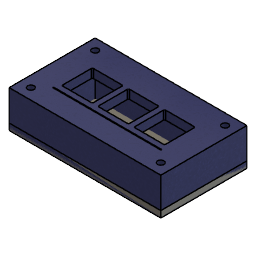
My case (Autodesk Fusion 360 design; units mm, degrees)
part number: 2026-08-28-17-32-42-272
Autodesk Fusion 360 part; units mm, degrees
sketch "Sketch1" plane through (0, 0, 0) normal (0, 1, 0) x (1, 0, 0)
  line L0 (0, 0) -> (49.4, 0)
  line L1 (49.4, 0) -> (49.4, -19.4)
  line L2 (49.4, -19.4) -> (0, -19.4)
  line L3 (0, -19.4) -> (0, 0)
  line L4 (-10, 10) -> (59.4, 10)
  line L5 (59.4, 10) -> (59.4, -29.4)
  line L6 (59.4, -29.4) -> (-10, -29.4)
  line L7 (-10, -29.4) -> (-10, 10)
  circle A0 centre (-5, 5) radius 1.45
  circle A1 centre (54.4, 5) radius 1.45
  circle A2 centre (54.4, -24.4) radius 1.45
  circle A3 centre (-5, -24.4) radius 1.45
  point P0 (-5, 5)
  point P1 (54.4, 5)
  point P2 (54.4, -24.4)
  point P3 (-5, -24.4)
  dimension "d1" = 19.4
  dimension "d2" = 49.4
  dimension "d3" = 39.4
  dimension "d4" = 69.4
  dimension "d5" = 5
  dimension "d6" = 5
  dimension "d7" = 5
  dimension "d8" = 5
  dimension "d9" = 5
  dimension "d10" = 5
  dimension "d11" = 2.9
  dimension "d12" = 2.9
  dimension "d13" = 2.9
  dimension "d14" = 2.9
  constraint horizontal L0
  constraint vertical L1
  constraint horizontal L2
  constraint vertical L3
  constraint coincident L0.start L3.end
  constraint horizontal L4
  constraint vertical L5
  constraint horizontal L6
  constraint vertical L7
  constraint coincident P0 A0.centre
  constraint coincident P1 A1.centre
  constraint coincident P2 A2.centre
  constraint coincident P3 A3.centre
  measures "d1" distance of L0.start L2.end
  measures "d2" distance of L0.start L0.end
  measures "d3" distance of L4.start L6.end
  measures "d4" distance of L4.start L4.end
  measures "d5" distance of L4 P1
  measures "d6" distance of L5 P1
  measures "d7" distance of L5 P2
  measures "d8" distance of L6 P2
  measures "d9" distance of L6 P3
  measures "d10" distance of L7 P3
  measures "d11" diameter of A0
  measures "d12" diameter of A1
  measures "d13" diameter of A2
  measures "d14" diameter of A3
extrude "Extrude1" add sketch "Sketch1" along normal blind 3 contours L0 L1 L2 L3 | L4 L5 L6 L7 makes body 1
extrude "Extrude2" add sketch "Sketch1" along normal blind 13 separate body makes body 2
sketch "plate-2026-08-28T13_17_58.150Z" plane through (0, 13, 0) normal (0, 1, 0) x (1, 0, 0)
  line L0 (1.7475, -2.525) -> (14.7475, -2.525)
  line L1 (1.7475, -16.525) -> (14.7475, -16.525)
  line L2 (1.2475, -3.025) -> (1.2475, -16.025)
  line L3 (15.2475, -3.025) -> (15.2475, -16.025)
  arc A0 (1.7475, -2.525) -> (1.2475, -3.025) centre (1.7475, -3.025) ccw
  arc A1 (15.2475, -3.025) -> (14.7475, -2.525) centre (14.7475, -3.025) ccw
  arc A2 (1.2475, -16.025) -> (1.7475, -16.525) centre (1.7475, -16.025) ccw
  arc A3 (14.7475, -16.525) -> (15.2475, -16.025) centre (14.7475, -16.025) ccw
  line L4 (18.2425, -2.525) -> (31.2425, -2.525)
  line L5 (18.2425, -16.525) -> (31.2425, -16.525)
  line L6 (17.7425, -3.025) -> (17.7425, -16.025)
  line L7 (31.7425, -3.025) -> (31.7425, -16.025)
  arc A4 (18.2425, -2.525) -> (17.7425, -3.025) centre (18.2425, -3.025) ccw
  arc A5 (31.7425, -3.025) -> (31.2425, -2.525) centre (31.2425, -3.025) ccw
  arc A6 (17.7425, -16.025) -> (18.2425, -16.525) centre (18.2425, -16.025) ccw
  arc A7 (31.2425, -16.525) -> (31.7425, -16.025) centre (31.2425, -16.025) ccw
  line L8 (34.7375, -2.525) -> (47.7375, -2.525)
  line L9 (34.7375, -16.525) -> (47.7375, -16.525)
  line L10 (34.2375, -3.025) -> (34.2375, -16.025)
  line L11 (48.2375, -3.025) -> (48.2375, -16.025)
  arc A8 (34.7375, -2.525) -> (34.2375, -3.025) centre (34.7375, -3.025) ccw
  arc A9 (48.2375, -3.025) -> (47.7375, -2.525) centre (47.7375, -3.025) ccw
  arc A10 (34.2375, -16.025) -> (34.7375, -16.525) centre (34.7375, -16.025) ccw
  arc A11 (47.7375, -16.525) -> (48.2375, -16.025) centre (47.7375, -16.025) ccw
  line L12 (0, -19.05) -> (49.485, -19.05)
  line L13 (0, 0) -> (49.485, 0)
  line L14 (0, -19.05) -> (0, 0)
  line L15 (49.485, -19.05) -> (49.485, 0)
extrude "Extrude3" add sketch "plate-2026-08-28T13_17_58.150Z" 1 faces at (32.9333, 13, 23.1528) along normal blind 4 on bodies 2 bodies 2
